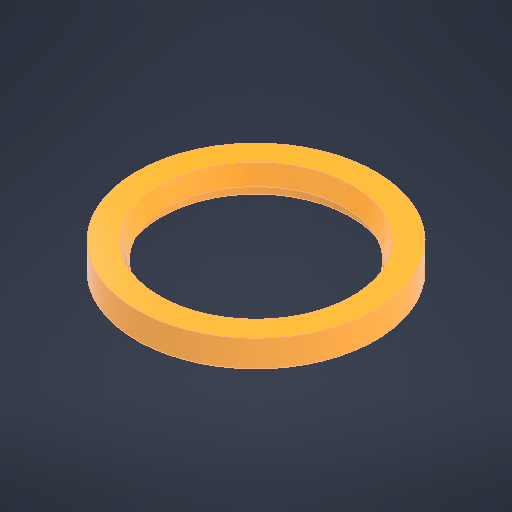
# Autodesk Inventor part: BASE_INFERIOR_FENOLICO
Saved by Autodesk Inventor 2025 (Build 290162010, 162A)
## iProperties
Created: 2024-07-24
Part Number: BASE_INFERIOR_FENOLICO
Material: Resina fenólica
Document SubType Name: Modeling
Designer: hansm
Density: 1.38 g/cm^3
Appearance: Suave - Naranja claro
Author: hansm
Autodesk Inventor part; units mm, degrees
ref_plane "YZ Plane" through (0, 0, 0) normal (1, 0, 0) x (0, 1, 0)
ref_plane "XZ Plane" through (0, 0, 0) normal (0, 1, 0) x (-1, 0, 0)
ref_plane "XY Plane" through (0, 0, 0) normal (0, 0, 1) x (1, 0, 0)
sketch "Boceto1" plane through (0, 0, 0) normal (0, 0, 1) x (1, 0, 0)
  line L0 (-36, 50.5) -> (-32, 50.5)
  line L1 (-32, 50.5) -> (-28.5, 50.5)
  line L2 (-36, 50.5) -> (-36, 58.5)
  line L3 (-36, 58.5) -> (-29, 58.5)
  line L4 (-29, 58.5) -> (-27, 53.5)
  line L5 (-27, 53.5) -> (-28.5, 53.5)
  line L6 (-28.5, 53.5) -> (-28.5, 50.5)
  line L7 (-36, 50.5) -> (-36, -0.0078) construction
  line L8 (0, -11.7094) -> (0, 70.2016) projected
  dimension "d12" = 4
  dimension "d21" = 3.5
  dimension "d22" = 8
  dimension "d23" = 50.5078
  dimension "d25" = 1.5
  dimension "d26" = 3
  dimension "d27" = 7
  constraints: 16 end point, 2 perpendicular, 2 vertical, 1 horizontal, 1 parallel
  measures "d12" distance of L0.start L0.end
  measures "d21" distance of L0.end L1.end
  measures "d22" distance of L0.start L2.end
  measures "d23" distance of L0.start L7.end
  measures "d25" distance of L4.end L5.end
  measures "d26" distance of L5.end L1.end
  measures "d27" distance of L2.end L3.end
revolve "Revolución1" add sketch "Boceto1" angle 360 about axis through (0, -10, 0) along (0, 1, 0)
